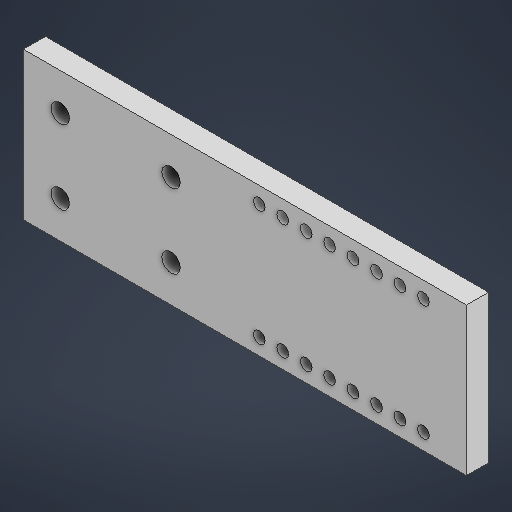
# Autodesk Inventor part: motor_bracket_base2
Saved by Autodesk Inventor 2026 (Build 300175050, 175E)
## iProperties
Created: 2025-11-11
Part Number: motor_bracket_base2
Material: Generic
Document SubType Name: Modeling
Designer: habbo
Density: 1 g/cm^3
Appearance: Default
Author: habbo
Autodesk Inventor part; units mm, degrees
ref_plane "YZ Plane" through (0, 0, 0) normal (1, 0, 0) x (0, 1, 0)
ref_plane "XZ Plane" through (0, 0, 0) normal (0, 1, 0) x (-1, 0, 0)
ref_plane "XY Plane" through (0, 0, 0) normal (0, 0, 1) x (1, 0, 0)
sketch "Sketch1" plane through (0, 0, 0) normal (0, 0, 1) x (1, 0, 0)
  line L0 (-60, -20) -> (60, -20)
  line L1 (60, -20) -> (60, 20)
  line L2 (60, 20) -> (-60, 20)
  line L3 (-60, 20) -> (-60, -20)
  line L4 (-60, -20) -> (60, 20) construction
  line L5 (60, -20) -> (-60, 20) construction
  circle A0 centre (42, -15.621) radius 1.5875
  circle A1 centre (22.95, -15.621) radius 1.5875
  circle A2 centre (3.9, -15.621) radius 1.5875
  circle A3 centre (42, 15.621) radius 1.5875
  circle A4 centre (22.95, 15.621) radius 1.5875
  circle A5 centre (3.9, 15.621) radius 1.5875
  circle A6 centre (-50, -10) radius 2.5
  circle A7 centre (-50, 10) radius 2.5
  circle A8 centre (10.25, -15.621) radius 1.5875
  circle A9 centre (16.6, -15.621) radius 1.5875
  circle A10 centre (29.3, -15.621) radius 1.5875
  circle A11 centre (35.65, -15.621) radius 1.5875
  line L6 (-5.5859, 0) -> (7.9995, 0) construction
  circle A12 centre (10.25, 15.621) radius 1.5875
  circle A13 centre (16.6, 15.621) radius 1.5875
  circle A14 centre (29.3, 15.621) radius 1.5875
  circle A15 centre (35.65, 15.621) radius 1.5875
  circle A16 centre (-20, -10) radius 2.5
  circle A17 centre (-20, 10) radius 2.5
  circle A18 centre (48.35, -15.621) radius 1.5875
  circle A19 centre (48.35, 15.621) radius 1.5875
  point P0 (0, 0)
  dimension "d0" = 120
  dimension "d1" = 40
  dimension "d4" = 3.175
  dimension "d5" = 3.175
  dimension "d6" = 3.175
  dimension "d7" = 3.175
  dimension "d8" = 3.175
  dimension "d9" = 3.175
  dimension "d10" = 31.242
  dimension "d11" = 19.05
  dimension "d12" = 19.05
  dimension "d13" = 18
  dimension "d16" = 5
  dimension "d17" = 5
  dimension "d21" = 10
  dimension "d26" = 4.379
  dimension "d29" = 3.175
  dimension "d30" = 3.175
  dimension "d31" = 3.175
  dimension "d32" = 3.175
  dimension "d33" = 6.35
  dimension "d34" = 6.35
  dimension "d35" = 6.35
  dimension "d36" = 6.35
  dimension "d39" = 5
  dimension "d40" = 5
  dimension "d41" = 30
  dimension "d42" = 3.175
  dimension "d43" = 6.35
  constraints: 20 centre point, 14 end point, 7 horizontal alignment, 6 vertical alignment, 4 symmetric about line, 2 horizontal, 2 midpoint, 2 parallel, 1 perpendicular, 4 other
  measures "d0" distance of L2.end L1.end
  measures "d1" distance of L1.end L0.end
  measures "d4" diameter of A0
  measures "d5" diameter of A1
  measures "d6" diameter of A2
  measures "d7" diameter of A3
  measures "d8" diameter of A4
  measures "d9" diameter of A5
  measures "d10" distance of A3.centre A0.centre
  measures "d11" distance of A1.centre A0.centre
  measures "d12" distance of A2.centre A1.centre
  measures "d13" distance from line of L1 A0.centre
  measures "d16" diameter of A6
  measures "d17" diameter of A7
  measures "d21" distance from line of A6.centre L3
  measures "d26" distance from line of L0 A0.centre
  measures "d29" diameter of A8
  measures "d30" diameter of A9
  measures "d31" diameter of A10
  measures "d32" diameter of A11
  measures "d33" distance of A8.centre A2.centre
  measures "d34" distance of A9.centre A8.centre
  measures "d35" distance of A1.centre A10.centre
  measures "d36" distance of A11.centre A10.centre
  measures "d39" diameter of A16
  measures "d40" diameter of A17
  measures "d41" distance of A17.centre A7.centre
  measures "d42" diameter of A18
  measures "d43" distance of A19.centre A3.centre
extrude "Extrusion4" add sketch "Sketch1" along normal mid plane 6
body "Solid4"
